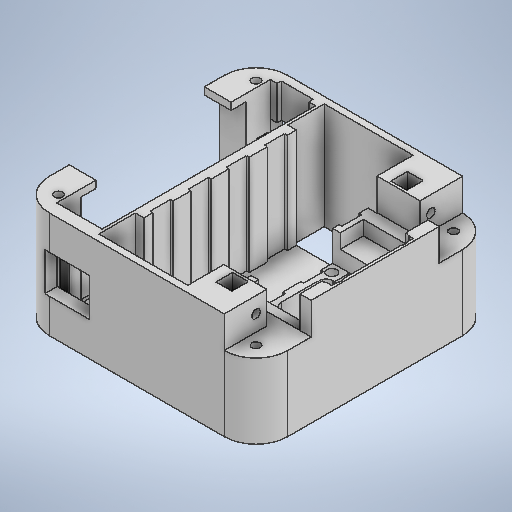
# Autodesk Inventor part: enclosure
Saved by Autodesk Inventor 2025 (Build 290162000, 162)
## iProperties
Created: 2025-10-18
Part Number: enclosure
Material: 一般
Document SubType Name: Modeling
Designer: sooo1
Density: 1 g/cm^3
Appearance: 既定
Author: sooo1
Autodesk Inventor part; units mm, degrees
ref_plane "YZ Plane" through (0, 0, 0) normal (1, 0, 0) x (0, 1, 0)
ref_plane "XZ Plane" through (0, 0, 0) normal (0, 1, 0) x (-1, 0, 0)
sketch "スケッチ1" plane through (0, 0, 0) normal (0, 1, 0) x (-1, 0, 0)
  line L0 (37.55, 37.55) -> (-37.55, 37.55)
  line L1 (-37.55, 37.55) -> (-37.55, -37.55)
  line L2 (-37.55, -37.55) -> (37.55, -37.55)
  line L3 (37.55, -37.55) -> (37.55, 37.55)
  line L4 (37.55, 37.55) -> (-37.55, -37.55) construction
  line L5 (-37.55, 37.55) -> (37.55, -37.55) construction
  line L6 (36.55, 36.55) -> (-36.55, 36.55)
  line L7 (-36.55, 36.55) -> (-36.55, -36.55)
  line L8 (-36.55, -36.55) -> (36.55, -36.55)
  line L9 (36.55, -36.55) -> (36.55, 36.55)
  line L10 (52.57, 0) -> (-52.57, 0) construction
  line L11 (0, -52.57) -> (0, 52.57) construction
  line L12 (14, -25) -> (-14, -25)
  line L13 (-14, -25) -> (-14, -35.5)
  line L14 (-14, -35.5) -> (14, -35.5)
  line L15 (14, -35.5) -> (14, -25)
  line L16 (14, -25) -> (-14, -35.5) construction
  line L17 (-14, -25) -> (14, -35.5) construction
  line L18 (0, 37.55) -> (0, -37.55) construction
  circle A0 centre (-13.68, -10.17) radius 1.6
  line L19 (14, -30.25) -> (-14, -30.25) construction
  line L20 (-11.15, 0) -> (-11.15, -24)
  line L21 (11.15, -24) -> (11.15, 0)
  line L22 (-11.15, 12.7) -> (-36.55, 12.7)
  line L23 (-36.55, 12.7) -> (-36.55, -12.7) construction
  line L24 (-36.55, -12.7) -> (-11.15, -12.7)
  line L25 (-11.15, -12.7) -> (-11.15, 12.7) construction
  line L26 (-11.15, 12.7) -> (-36.55, -12.7) construction
  line L27 (-36.55, 12.7) -> (-11.15, -12.7) construction
  line L28 (-13.68, 10.17) -> (-34.02, 10.17) construction
  line L29 (-34.02, 10.17) -> (-34.02, -10.17) construction
  line L30 (-34.02, -10.17) -> (-13.68, -10.17) construction
  line L31 (-13.68, -10.17) -> (-13.68, 10.17) construction
  line L32 (-13.68, 10.17) -> (-34.02, -10.17) construction
  line L33 (-34.02, 10.17) -> (-13.68, -10.17) construction
  circle A1 centre (-13.68, 10.17) radius 1.6
  circle A2 centre (-34.02, 10.17) radius 1.6
  circle A3 centre (-34.02, -10.17) radius 1.6
  line L34 (11.15, 0) -> (-11.15, 0) construction
  line L35 (11.15, -24) -> (-11.15, -24)
  line L36 (8.8, -24) -> (-8.8, -24) construction
  line L37 (-8.8, -24) -> (-8.8, -27)
  line L38 (-8.8, -27) -> (8.8, -27)
  line L39 (8.8, -27) -> (8.8, -24)
  line L40 (8.8, -24) -> (-8.8, -27) construction
  line L41 (-8.8, -24) -> (8.8, -27) construction
  line L42 (11.15, -3) -> (12, -3)
  line L43 (12, -3) -> (12, -9)
  line L44 (12, -9) -> (11.15, -9)
  line L45 (11.15, -12) -> (-11.15, -12) construction
  line L46 (12, -6) -> (-12, -6) construction
  line L47 (11.15, -21) -> (12, -21)
  line L48 (12, -21) -> (12, -15)
  line L49 (12, -15) -> (11.15, -15)
  line L50 (-11.15, -3) -> (-12, -3)
  line L51 (-12, -3) -> (-12, -9)
  line L52 (-12, -9) -> (-11.15, -9)
  line L53 (-12, -15) -> (-11.15, -15)
  line L54 (-12, -21) -> (-12, -15)
  line L55 (-11.15, -21) -> (-12, -21)
  line L56 (14, 25) -> (-14, 25)
  line L57 (-14, 25) -> (-14, 35.5)
  line L58 (-14, 35.5) -> (14, 35.5)
  line L59 (14, 35.5) -> (14, 25)
  line L60 (-11.15, 0) -> (-11.15, 24)
  line L61 (11.15, 24) -> (11.15, 0)
  line L62 (11.15, 24) -> (-11.15, 24)
  line L63 (8.8, 24) -> (-8.8, 24) construction
  line L64 (-8.8, 24) -> (-8.8, 27)
  line L65 (-8.8, 27) -> (8.8, 27)
  line L66 (8.8, 27) -> (8.8, 24)
  line L67 (11.15, 3) -> (12, 3)
  line L68 (12, 3) -> (12, 9)
  line L69 (12, 9) -> (11.15, 9)
  line L70 (12, 15) -> (11.15, 15)
  line L71 (12, 21) -> (12, 15)
  line L72 (11.15, 21) -> (12, 21)
  line L73 (-12, 3) -> (-12, 9)
  line L74 (-11.15, 3) -> (-12, 3)
  line L75 (-12, 9) -> (-11.15, 9)
  line L76 (-12, 21) -> (-12, 15)
  line L77 (-12, 15) -> (-11.15, 15)
  line L78 (-11.15, 21) -> (-12, 21)
  line L79 (15, 33.5) -> (29, 33.5)
  line L80 (29, 33.5) -> (29, -33.5)
  line L81 (29, -33.5) -> (15, -33.5)
  line L82 (15, -33.5) -> (15, 33.5)
  line L83 (15, 33.5) -> (29, -33.5) construction
  line L84 (29, 33.5) -> (15, -33.5) construction
  line L85 (-33.85, 20) -> (-13.85, 20)
  line L86 (-13.85, 20) -> (-13.85, -20)
  line L87 (-13.85, -20) -> (-33.85, -20)
  line L88 (-33.85, -20) -> (-33.85, 20)
  line L89 (-33.85, 20) -> (-13.85, -20) construction
  line L90 (-13.85, 20) -> (-33.85, -20) construction
  line L91 (37.55, 25.5) -> (15, 25.5) construction
  circle A4 centre (-21, -30.25) radius 3.1
  line L92 (-21, -37.55) -> (-21, 37.55) construction
  circle A5 centre (-21, 30.25) radius 3.1
  circle A6 centre (21, -30.25) radius 3.1
  circle A7 centre (21, 30.25) radius 3.1
  circle A8 centre (-21, -30.25) radius 4.1
  circle A9 centre (-21, 30.25) radius 4.1
  circle A10 centre (21, -30.25) radius 4.1
  circle A11 centre (21, 30.25) radius 4.1
  circle A12 centre (33, 0) radius 2.6
  circle A13 centre (33, 0) radius 3.5
  circle A14 centre (-33, 0) radius 2.6
  circle A15 centre (-33, 0) radius 3.5
  line L93 (-27.85, 4) -> (-19.85, 4)
  line L94 (-19.85, 4) -> (-19.85, -4)
  line L95 (-19.85, -4) -> (-27.85, -4)
  line L96 (-27.85, -4) -> (-27.85, 4)
  line L97 (-27.85, 4) -> (-19.85, -4) construction
  line L98 (-19.85, 4) -> (-27.85, -4) construction
  line L99 (26, -34) -> (18, -34)
  line L100 (18, -34) -> (18, -33.5)
  line L101 (18, -33.5) -> (26, -33.5) construction
  line L102 (26, -33.5) -> (26, -34)
  line L103 (26, -34) -> (18, -33.5) construction
  line L104 (18, -34) -> (26, -33.5) construction
  line L105 (22, -33.5) -> (22, 33.5) construction
  line L106 (-11.15, 24) -> (-11.15, 25)
  line L107 (11.15, 24) -> (11.15, 25)
  line L108 (11.15, -24) -> (11.15, -25)
  line L109 (-11.15, -24) -> (-11.15, -25)
  line L110 (14, 25) -> (14, 24)
  line L111 (14, 24) -> (11.15, 24)
  line L112 (-11.15, 24) -> (-14, 24)
  line L113 (-14, 24) -> (-14, 25)
  line L114 (14, -25) -> (14, -24)
  line L115 (14, -24) -> (11.15, -24)
  line L116 (-11.15, -24) -> (-14, -24)
  line L117 (-14, -24) -> (-14, -25)
  line L118 (-11.15, 8.17) -> (-36.55, 8.17)
  line L119 (-11.15, -8.17) -> (-36.55, -8.17)
  line L120 (-11.15, 13) -> (-36.55, 13)
  line L121 (-11.15, -13) -> (-36.55, -13)
  line L122 (-16.65, 13) -> (-16.65, -13)
  line L123 (-29.55, 13) -> (-29.55, -13)
  line L124 (-36.55, 13) -> (-37.55, 13)
  line L125 (-36.55, -13) -> (-37.55, -13)
  line L126 (-27.85, 4) -> (-27.85, 13)
  line L127 (-27.85, -4) -> (-27.85, -13)
  point P0 (0, 0)
  point P1 (0, -30.25)
  point P2 (-23.85, 0)
  point P3 (0, -25.5)
  point P4 (0, 0)
  point P5 (0, -6)
  point P6 (-12, 6)
  point P7 (12, 6)
  point P8 (22, 0)
  point P9 (-23.85, 0)
  point P10 (22, -33.75)
  point P11 (-29.55, 0.5895)
  point P12 (-29.55, -0.5895)
  point P13 (-29.55, -8.17)
  point P14 (-29.55, 8.17)
  point P15 (-27.85, 12.7)
  point P16 (-29.55, 12.7)
  point P17 (-16.65, -8.17)
  point P18 (-13.85, -8.17)
  point P19 (-13.85, 8.17)
  point P20 (-16.65, 8.17)
  point P21 (-33.85, 8.17)
  point P22 (-33.85, -8.17)
  point P23 (-29.55, -12.7)
  point P24 (-16.65, -12.7)
  point P25 (-16.65, 12.7)
  dimension "d1" = 1
  dimension "d2" = 10.5
  dimension "d3" = 28
  dimension "d5" = 3.2
  dimension "d11" = 25.4
  dimension "d12" = 20.34
  dimension "d15" = 360
  dimension "d18" = 22.3
  dimension "d19" = 17.6
  dimension "d20" = 27
  dimension "d21" = 24
  dimension "d22" = 1
  dimension "d25" = 24
  dimension "d26" = 12
  dimension "d27" = 6
  dimension "d32" = 67
  dimension "d33" = 14
  dimension "d34" = 1
  dimension "d35" = 40
  dimension "d36" = 20
  dimension "d41" = 8
  dimension "d47" = 6.2
  dimension "d48" = 7
  dimension "d49" = 1
  dimension "d54" = 5.2
  dimension "d55" = 7
  dimension "d56" = 33
  dimension "d86" = 8
  dimension "d110" = 8
  dimension "d111" = 0.5
  dimension "d177" = 8.17
  dimension "d178" = 8.17
  dimension "d179" = 0.3
  dimension "d180" = 0.3
  dimension "d181" = 7
  dimension "d182" = 5.5
  constraints: 252 end point, 48 symmetric about line, 45 point on line, 31 perpendicular, 30 midpoint, 22 parallel, 16 centre point, 11 horizontal, 8 collinear, 5 coincident, 3 equal length, 1 vertical, 20 other
  measures "d1" distance between parallel lines of L0 L6
  measures "d2" distance of L14.end L12.start
  measures "d3" distance of L13.end L14.end
  measures "d5" diameter of A0
  measures "d11" distance of L24.end L22.start
  measures "d12" distance of L30.end L28.start
  measures "d18" distance between parallel lines of L20 L21
  measures "d19" distance of L37.end L38.end
  measures "d20" distance between parallel lines of L34 L38
  measures "d21" distance of L21.start L21.end
  measures "d22" distance between parallel lines of L12 L35
  measures "d25" distance of L46.start L46.end
  measures "d26" diameter of L46 L45
  measures "d27" distance of L42.end L43.end
  measures "d32" distance of L79.end L80.end
  measures "d33" distance of L79.start L79.end
  measures "d34" distance between parallel lines of L82 L59
  measures "d35" distance of L87.end L85.start
  measures "d36" distance of L85.start L85.end
  measures "d41" distance between parallel lines of L79 L91
  measures "d47" diameter of A4
  measures "d48" distance between parallel lines of L13 L92
  measures "d49" radial gap between concentric circles of A4 A8
  measures "d54" diameter of A12
  measures "d55" diameter of A13
  measures "d56" distance from line of L11 A12.centre
  measures "d86" distance of L95.end L93.start
  measures "d110" distance of L99.start L99.end
  measures "d111" distance of L101.end L99.start
  measures "d177" distance between parallel lines of L10 L118
  measures "d178" distance between parallel lines of L119 L10
  measures "d179" distance between parallel lines of L22 L120
  measures "d180" distance between parallel lines of L121 L24
  measures "d181" distance between parallel lines of L23 L123
  measures "d182" distance between parallel lines of L25 L122
extrude "押し出し3" add sketch "スケッチ1" along normal blind 33.5 contours L3 L2 L1 L125 L7 L8 L9 L6 L124 L0 | L124 L7 L125 L1 | L120 L88 L22 L7 | L7 L6 L9 L8 L121 L88 L87 L86 L20 L53 L54 L55 L116 L117 L13 L14 L15 L114 L115 L21 L47 L48 L49 L44 L43 L42 L61 L67 L68 L69 L70 L71 L72 L111 L110 L59 L58 L57 L113 L112 L60 L78 L76 L77 L120 L85 | L7 L24 L88 L121 | L22 L88 A2 L118 L7 | L120 L123 L22 L88 | L88 L85 L86 L120 | L7 L119 L88 A3 L24 | L121 L86 L87 L88 | L88 L24 L123 L121 | L118 L88 A15 L119 L7 | L22 L123 L118 L88 A2 | L120 L126 L22 L123 | L88 A3 L119 L123 L24 | L123 L24 L127 L121 | L118 L123 A15 L88 | L22 L126 L118 L123 | L88 A2 | A2 L88 | L120 L122 L22 L126 | L88 A15 L123 L119 | L123 L119 L127 L24 | L88 A3 | A3 L88 | L127 L24 L122 L121 | A15 L123 L88 A14 | L88 A14 A15 | L118 L126 L96 L127 L119 L123 A15 | L22 L122 L118 L126 | L120 L60 L22 L86 | L86 L22 L122 L120 | L127 L119 L122 L24 | L121 L122 L24 L86 | L86 L24 L20 L121 | A14 L88 | L88 A14 | A15 L123 | L118 L122 L119 L127 L95 L94 L93 L126 | L22 L86 A1 L118 L122 | L22 L60 L75 L73 L118 L86 A1 | L60 L62 L61 L21 L35 L20 | L122 L119 L86 A0 L24 | L86 A0 L119 L51 L52 L20 L24 | L118 L86 L119 L122 | L93 L94 L95 L96 | L86 A1 | A1 L86 | L77 L76 L78 L60 | L86 A0 | A0 L86 | L20 L55 L54 L53 | L118 L73 L74 L60 L20 L50 L51 L119 L86 | L60 L118 L73 L75 | L52 L51 L119 L20 | L118 L60 L74 L73 | L106 L56 L64 L62 | L112 L113 L56 L106 | L51 L50 L20 L119 | L35 L37 L12 L109 | L109 L12 L117 L116 | L64 L56 L66 L62 | L56 L57 L58 L59 L66 L65 L64 | L35 L39 L12 L37 | L12 L37 L38 L39 L15 L14 L13 | L66 L56 L107 L62 | L64 L65 L66 L56 | L35 L108 L12 L39 | L12 L39 L38 L37 | L107 L56 L110 L111 | L115 L114 L12 L108 | L72 L71 L70 L61 | L21 L49 L48 L47 | L69 L68 L67 L61 | L21 L42 L43 L44 | L79 A11 L80 L81 A10 L82 | A11 L79 | L79 A11 | L81 A10 L99 L100 | A10 L81 | L81 A10 L99 | L81 L102 L99 A10 | L99 A10 | A4 | A5 | A6 | A7 | A8 | A9 | A12 | A13
fillet "フィレット1" radius 10 4 edges at (37.55, 16.75, 37.55) (37.55, 16.75, -37.55) (-37.55, 16.75, -37.55) (-37.55, 16.75, 37.55)
extrude "押し出し11" cut sketch "スケッチ1" along normal through all contours L56 L57 L58 L59 L66 L65 L64 | L12 L37 L38 L39 L15 L14 L13 | L64 L65 L66 L56 | L12 L39 L38 L37
extrude "押し出し12" cut sketch "スケッチ1" along normal blind 1.5 contours A4 | A5 | A6 | A7
extrude "押し出し13" cut sketch "スケッチ1" along normal blind 1.5 contours A14 L88 | L88 A14 | A12
sketch "スケッチ5" plane through (0, 0, 0) normal (0, 1, 0) x (-1, 0, 0)
  line L0 (-12, 9) -> (-11.15, 9) projected
  line L1 (-11.15, 0) -> (-11.15, 24) projected
  line L2 (-12, 3) -> (-12, 9) projected
  line L3 (-11.15, 3) -> (-12, 3) projected
  line L4 (-12, 15) -> (-11.15, 15) projected
  line L5 (-12, 21) -> (-12, 15) projected
  line L6 (11.15, 3) -> (12, 3) projected
  line L7 (-11.15, 21) -> (-12, 21) projected
  line L8 (11.15, 21) -> (12, 21) projected
  line L9 (11.15, 24) -> (-11.15, 24) projected
  line L10 (-8.8, 24) -> (-8.8, 27) projected
  line L11 (8.8, 24) -> (-8.8, 24) construction
  line L12 (8.8, 27) -> (8.8, 24) projected
  line L13 (-8.8, 27) -> (8.8, 27) projected
  line L14 (11.15, 0) -> (-11.15, 0) construction
  line L15 (11.15, -12) -> (-11.15, -12) construction
  line L16 (12, -9) -> (11.15, -9) projected
  line L17 (11.15, -3) -> (12, -3) projected
  line L18 (12, -3) -> (12, -9) projected
  line L19 (12, -6) -> (-12, -6) construction
  line L20 (-12, -9) -> (-11.15, -9) projected
  line L21 (-12, -3) -> (-12, -9) projected
  line L22 (-11.15, -3) -> (-12, -3) projected
  line L23 (-11.15, -12.7) -> (-11.15, 12.7) construction
  line L24 (-11.15, 0) -> (-11.15, -24) projected
  line L25 (11.15, -24) -> (11.15, 0) projected
  line L26 (12, -15) -> (11.15, -15) projected
  line L27 (12, -21) -> (12, -15) projected
  line L28 (12, 9) -> (11.15, 9) projected
  line L29 (12, 3) -> (12, 9) projected
  line L30 (12, 15) -> (11.15, 15) projected
  line L31 (12, 21) -> (12, 15) projected
  line L32 (11.15, 24) -> (11.15, 0) projected
  line L33 (11.15, -24) -> (-11.15, -24) projected
  line L34 (8.8, -24) -> (-8.8, -24) construction
  line L35 (-12, -15) -> (-11.15, -15) projected
  line L36 (-12, -21) -> (-12, -15) projected
  line L37 (-11.15, -21) -> (-12, -21) projected
  line L38 (11.15, -21) -> (12, -21) projected
  line L39 (-8.8, -27) -> (8.8, -27) projected
  line L40 (-8.8, -24) -> (-8.8, -27) projected
  line L41 (8.8, -27) -> (8.8, -24) projected
  line L42 (-11.15, -14.85) -> (-12.15, -14.85)
  line L43 (-12.15, -14.85) -> (-12.15, -21.15)
  line L44 (-12.15, -21.15) -> (-11.15, -21.15)
  line L45 (-11.15, -9.15) -> (-12.15, -9.15)
  line L46 (-12.15, -9.15) -> (-12.15, -2.85)
  line L47 (-12.15, -2.85) -> (-11.15, -2.85)
  line L48 (11.15, -14.85) -> (12.15, -14.85)
  line L49 (12.15, -14.85) -> (12.15, -21.15)
  line L50 (12.15, -21.15) -> (11.15, -21.15)
  line L51 (11.15, -9.15) -> (12.15, -9.15)
  line L52 (12.15, -9.15) -> (12.15, -2.85)
  line L53 (12.15, -2.85) -> (11.15, -2.85)
  line L54 (-11.15, 9.15) -> (-12.15, 9.15)
  line L55 (-12.15, 9.15) -> (-12.15, 2.85)
  line L56 (-12.15, 2.85) -> (-11.15, 2.85)
  line L57 (-11.15, 14.85) -> (-12.15, 14.85)
  line L58 (-12.15, 14.85) -> (-12.15, 21.15)
  line L59 (-12.15, 21.15) -> (-11.15, 21.15)
  line L60 (11.15, 14.85) -> (12.15, 14.85)
  line L61 (12.15, 14.85) -> (12.15, 21.15)
  line L62 (12.15, 21.15) -> (11.15, 21.15)
  line L63 (-11.3, -24.15) -> (-11.3, 0)
  line L64 (-11.3, 0) -> (-11.3, 24.15)
  line L65 (-11.3, 24.15) -> (11.3, 24.15)
  line L66 (11.3, 24.15) -> (11.3, 0)
  line L67 (11.3, 0) -> (11.3, -24.15)
  line L68 (11.3, -24.15) -> (-11.3, -24.15)
  line L69 (8.95, 27.15) -> (8.95, 23.85)
  line L70 (8.95, 23.85) -> (-8.95, 23.85)
  line L71 (-8.95, 23.85) -> (-8.95, 27.15)
  line L72 (-8.95, 27.15) -> (8.95, 27.15)
  line L73 (8.95, -27.15) -> (-8.95, -27.15)
  line L74 (-8.95, -27.15) -> (-8.95, -23.85)
  line L75 (-8.95, -23.85) -> (8.95, -23.85)
  line L76 (8.95, -23.85) -> (8.95, -27.15)
  line L77 (11.15, 9.15) -> (12.15, 9.15)
  line L78 (12.15, 9.15) -> (12.15, 2.85)
  line L79 (12.15, 2.85) -> (11.15, 2.85)
  point P0 (0, 0)
  point P1 (0, 0)
  point P2 (-12, 6)
  point P3 (12, 6)
  point P4 (0, -6)
  point P5 (0, 0)
  point P6 (-11.3, -14.85)
  point P7 (-11.3, -21.15)
  point P8 (-8.95, -24.15)
  point P9 (8.95, -24.15)
  point P10 (11.3, -21.15)
  point P11 (11.3, -14.85)
  point P12 (11.3, -9.15)
  point P13 (11.3, -2.85)
  point P14 (11.3, 2.85)
  point P15 (11.3, 9.15)
  point P16 (11.3, 14.85)
  point P17 (11.3, 21.15)
  point P18 (8.95, 24.15)
  point P19 (-8.95, 24.15)
  point P20 (-11.3, 21.15)
  point P21 (-11.3, 14.85)
  point P22 (-11.3, 9.15)
  point P23 (-11.3, 2.85)
  point P24 (-11.3, -2.85)
  point P25 (-11.3, -9.15)
  dimension "d73" = 0.15
  dimension "d74" = 0.15
  dimension "d75" = 0.15
  dimension "d76" = 0.15
  dimension "d77" = 0.15
  dimension "d78" = 0.15
  dimension "d79" = 0.15
  dimension "d80" = 0.15
  dimension "d81" = 0.15
  dimension "d82" = 0.15
  dimension "d83" = 0.15
  constraints: 76 end point, 27 other
  measures "d73" distance between parallel lines of L24 L63
  measures "d74" distance between parallel lines of L36 L43
  measures "d75" distance between parallel lines of L39 L73
  measures "d76" distance between parallel lines of L21 L46
  measures "d77" distance between parallel lines of L2 L55
  measures "d78" distance between parallel lines of L5 L58
  measures "d79" distance between parallel lines of L13 L72
  measures "d80" distance between parallel lines of L61 L31
  measures "d81" distance between parallel lines of L18 L52
  measures "d82" distance between parallel lines of L27 L49
  measures "d83" distance between parallel lines of L29 L78
extrude "押し出し14" cut sketch "スケッチ5" against normal blind 31.5 from surface at 33.5
sketch "スケッチ6" plane through (0, 0, 0) normal (0, 1, 0) x (-1, 0, 0)
  line L0 (-11.15, 12.7) -> (-36.55, 12.7) projected
  circle A0 centre (-13.68, 10.17) radius 1.6 projected
  line L1 (-11.15, 0) -> (-11.15, 24) projected
  line L2 (-11.15, 0) -> (-11.15, -24) projected
  line L3 (-36.55, -12.7) -> (-11.15, -12.7) projected
  line L4 (-36.55, 12.7) -> (-36.55, -12.7) projected
  circle A1 centre (-34.02, -10.17) radius 1.6 projected
  circle A2 centre (-34.02, 10.17) radius 1.6 projected
  circle A3 centre (-13.68, -10.17) radius 1.6 projected
  line L5 (-11.15, 12.85) -> (-36.7, 12.85)
  line L6 (-36.7, 12.85) -> (-36.7, -12.85)
  line L7 (-36.7, -12.85) -> (-11.15, -12.85)
  circle A4 centre (-13.68, 10.17) radius 3
  circle A5 centre (-34.02, 10.17) radius 3
  circle A6 centre (-13.68, -10.17) radius 3
  circle A7 centre (-34.02, -10.17) radius 3
  line L8 (-11.15, 12.85) -> (-11.15, -12.85)
  line L9 (-12, 9) -> (-11.15, 9) projected
  line L10 (-11.15, 3) -> (-12, 3) projected
  line L11 (-11.15, -3) -> (-12, -3) projected
  line L12 (-12, -9) -> (-11.15, -9) projected
  line L13 (-11.15, -12.7) -> (-11.15, 12.7) projected
  line L14 (-36.55, 36.55) -> (-36.55, -36.55) projected
  line L15 (-36.55, 12.7) -> (-36.55, 12.85)
  line L16 (-36.55, -12.7) -> (-37.55, -12.85)
  line L17 (-37.55, 27.55) -> (-37.55, -27.55) projected
  line L18 (-11.15, -8.17) -> (-36.55, -8.17) projected
  line L19 (-11.15, 8.17) -> (-36.55, 8.17) projected
  line L20 (-36.55, 8.17) -> (-36.7, 8.17)
  line L21 (-36.55, -8.17) -> (-36.7, -8.17)
  point P0 (0, 0)
  point P1 (-36.7, -11.5182)
  point P2 (-36.7, -8.8218)
  point P3 (-32.6718, -12.85)
  point P4 (-35.3682, -12.85)
  point P5 (-36.7, 8.8218)
  point P6 (-36.7, 11.5182)
  point P7 (-35.3682, 12.85)
  point P8 (-32.6718, 12.85)
  point P9 (-36.55, -12.85)
  point P10 (-36.55, -11.7822)
  point P11 (-35.6322, -12.7)
  point P12 (-36.55, -12.7)
  point P13 (-36.4, -10.6381)
  point P14 (-36.4, -9.7019)
  point P15 (-36.4, 9.7019)
  point P16 (-36.4, 10.6381)
  point P17 (-36.55, 12.7)
  point P18 (-35.6322, 12.7)
  point P19 (-36.55, 11.7822)
  dimension "d89" = 0.15
  dimension "d92" = 6
  constraints: 14 end point, 6 point on line, 4 centre point, 3 equal radius, 3 perpendicular, 1 horizontal, 9 other
  measures "d89" distance between parallel lines of L0 L5
  measures "d92" diameter of A4
extrude "押し出し16" cut sketch "スケッチ6" against normal blind 19.5 from surface at 33.5 contours L1 A4 L0 | L0 A4 L5 L1 | A4 L1 L19 L0 | L0 A4 L5 | A4 L19 A5 L0 | L0 A5 L5 A4 | A5 L19 L4 L0 | L0 A5 L5 | L19 A4 | A4 L19 L1 L2 L18 A6 A7 L4 A5 | L1 L19 A4 | A5 L4 L0 | L0 L14 L5 A5 | L5 A5 | A5 L19 | L4 A5 L6 L5 L14 | L4 A5 L6 | L19 L4 A5 | L4 L20 L6 A5 | L6 A5 | L4 L21 L6 L20 | L18 A7 L4 | L4 A7 L6 L21 | A7 L18 L3 L4 | L4 A7 L6 | A7 L18 | L2 A6 L18 | A7 L3 L4 | L4 L16 L6 A7 | L6 A7 | L18 A6 L3 A7 | L2 A6 L3 L18 | L18 A6 | L3 A7 L7 L14 | L14 L7 L6 L16 | L3 A7 L7 | L3 A6 L7 A7 | L7 A7 | L3 A6 L7 | L2 L3 A6 | L3 L2 L7 A6 | A0 | A1 | A2 | A3
extrude "押し出し15" cut sketch "スケッチ1" along normal through all contours L88 A2 | A2 L88 | L88 A3 | A3 L88 | L93 L94 L95 L96 | L86 A1 | A1 L86 | L86 A0 | A0 L86
extrude "押し出し17" cut sketch "スケッチ6" along normal blind 4 contours A5 L19 L4 L0 | L0 A5 L5 | L5 A5 | A5 L19 | L4 A5 L6 | L6 A5 | A7 L18 L3 L4 | L4 A7 L6 | A7 L18 | L6 A7 | L3 A7 L7 | L7 A7 | A1 | A2
sketch "スケッチ7" plane through (0, 0, 0) normal (0, 1, 0) x (-1, 0, 0)
  line L0 (-33.85, 20) -> (-13.85, 20) projected
  line L1 (-13.85, 20) -> (-13.85, -20) projected
  line L2 (-33.85, -20) -> (-33.85, 20) projected
  line L3 (-13.85, -20) -> (-33.85, -20) projected
  line L4 (-13.7, 20.15) -> (-34, 20.15)
  line L5 (-34, 20.15) -> (-34, -20.15)
  line L6 (-34, -20.15) -> (-13.7, -20.15)
  line L7 (-13.7, -20.15) -> (-13.7, 20.15)
  point P0 (0, 0)
  dimension "d95" = 0.15
  constraints: 8 end point, 3 other
  measures "d95" distance between parallel lines of L0 L4
extrude "押し出し18" cut sketch "スケッチ7" against normal blind 14.5 from surface at 33.5 contours L0 L1 L3 L2 | L7 L6 L5 L4
sketch "スケッチ9" plane through (0, 0, 0) normal (0, 1, 0) x (-1, 0, 0)
  line L0 (29, 33.5) -> (29, -33.5) projected
  line L1 (29, -33.5) -> (15, -33.5) projected
  line L2 (15, -33.5) -> (15, 33.5) projected
  line L3 (15, 33.5) -> (29, 33.5) projected
  line L4 (29.15, -33.65) -> (29.15, 33.65)
  line L5 (29.15, 33.65) -> (14.85, 33.65)
  line L6 (14.85, 33.65) -> (14.85, -33.65)
  line L7 (14.85, -33.65) -> (29.15, -33.65)
  line L8 (15, -33.5) -> (15, -33.65)
  line L9 (15, 33.5) -> (15, 33.65)
  line L10 (26, -33.5) -> (26, -34) projected
  line L11 (26, -34) -> (18, -34) projected
  line L12 (18, -34) -> (18, -33.5) projected
  line L13 (16, -33.5) -> (16, -36)
  line L14 (16, -36) -> (28, -36)
  line L15 (28, -36) -> (28, -33.5)
  line L16 (28, -36) -> (28, -39.9042)
  line L17 (28, -39.9042) -> (16, -39.9042)
  line L18 (16, -39.9042) -> (16, -36)
  line L19 (17, -33.5) -> (17, -35)
  line L20 (17, -35) -> (27, -35)
  line L21 (27, -35) -> (27, -33.5)
  point P0 (0, 0)
  point P1 (22, -33.5)
  point P2 (18, -33.65)
  point P3 (26, -33.65)
  point P4 (17, -33.65)
  point P5 (27, -33.65)
  dimension "d109" = 0.15
  dimension "d113" = 12
  dimension "d116" = 10
  constraints: 30 end point, 3 point on line, 2 perpendicular, 2 vertical, 1 midpoint, 7 other
  measures "d109" distance from line of point (22, -33.5) L7
  measures "d113" distance of L13.end L14.end
  measures "d116" distance of L19.end L20.end
extrude "押し出し21" cut sketch "スケッチ9" against normal blind 31.25 from surface at 33.5 contours L3 L9 L5 L4 L7 L15 L1 L0 | L0 L1 L2 L3 | L2 L8 L7 L6 L5 L9 | L15 L7 L21 L1 | L1 L13 L7 L8 | L21 L7 L10 L1 | L1 L19 L7 L13 | L10 L7 L12 L1 | L21 L20 L19 L7 L12 L11 L10 | L1 L12 L7 L19 | L10 L11 L12 L7
sketch "スケッチ8" plane through (0, 0, 0) normal (1, 0, 0) x (0, 1, 0)
  line L0 (-10.4294, 0) -> (62.5761, 0) construction
  line L1 (0, -52.2157) -> (0, 71.794) construction
  line L2 (30.25, -33.5) -> (3.25, -33.5)
  line L3 (3.25, -33.5) -> (3.25, 33.5)
  line L4 (3.25, 33.5) -> (30.25, 33.5)
  line L5 (30.25, 33.5) -> (30.25, -33.5)
  line L6 (30.25, -33.5) -> (3.25, 33.5) construction
  line L7 (3.25, -33.5) -> (30.25, 33.5) construction
  line L8 (31.25, -34.5) -> (2.25, -34.5)
  line L9 (2.25, -34.5) -> (2.25, 34.5)
  line L10 (2.25, 34.5) -> (31.25, 34.5)
  line L11 (31.25, 34.5) -> (31.25, -34.5)
  line L12 (20.75, 33.5) -> (12.75, 33.5) construction
  line L13 (12.75, 33.5) -> (12.75, 34)
  line L14 (12.75, 34) -> (20.75, 34)
  line L15 (20.75, 34) -> (20.75, 33.5)
  line L16 (20.75, 33.5) -> (12.75, 34) construction
  line L17 (12.75, 33.5) -> (20.75, 34) construction
  line L18 (16.75, -33.5) -> (16.75, 33.5) construction
  line L19 (52.1468, -21.2895) -> (31.25, -21.2895)
  line L20 (31.25, -21.2895) -> (31.25, 21.2895) construction
  line L21 (31.25, 21.2895) -> (52.1468, 21.2895)
  line L22 (52.1468, 21.2895) -> (52.1468, -21.2895)
  line L23 (52.1468, -21.2895) -> (31.25, 21.2895) construction
  line L24 (31.25, -21.2895) -> (52.1468, 21.2895) construction
  line L25 (22.75, 33.5) -> (10.75, 33.5) construction
  line L26 (10.75, 33.5) -> (10.75, 54.0784)
  line L27 (10.75, 54.0784) -> (22.75, 54.0784)
  line L28 (22.75, 54.0784) -> (22.75, 33.5)
  line L29 (22.75, 33.5) -> (10.75, 54.0784) construction
  line L30 (10.75, 33.5) -> (22.75, 54.0784) construction
  line L31 (31.25, -26) -> (2.25, -26)
  line L32 (31.25, 26) -> (2.25, 26)
  point P0 (0, 0)
  point P1 (16.75, 0)
  point P2 (16.75, 33.75)
  point P3 (41.6984, 0)
  point P4 (16.75, 43.7892)
  point P5 (10.75, 34.5)
  point P6 (22.75, 34.5)
  point P7 (30.25, 26)
  point P8 (3.25, 26)
  point P9 (3.25, -26)
  point P10 (30.25, -26)
  dimension "d98" = 27
  dimension "d99" = 67
  dimension "d100" = 1
  dimension "d101" = 0.5
  dimension "d102" = 8
  dimension "d103" = 16.75
  dimension "d106" = 12
  dimension "d117" = 26
  constraints: 62 end point, 10 midpoint, 10 parallel, 7 perpendicular, 6 point on line, 4 horizontal, 3 collinear, 2 symmetric about line, 3 other
  measures "d98" distance of L2.start L2.end
  measures "d99" distance of L4.end L2.start
  measures "d100" distance between parallel lines of L2 L8
  measures "d101" distance of L14.end L12.start
  measures "d102" distance of L13.end L14.end
  measures "d103" distance between parallel lines of L1 L18
  measures "d106" distance of L26.end L27.end
  measures "d117" distance between parallel lines of L31 L0
extrude "押し出し22" cut sketch "スケッチ8" against normal blind 31.25 from surface at -29.15 contours L31 L3 L32 L5 | L5 L32 L11 L31 | L11 L21 L22 L19
sketch "スケッチ10" plane through (0, 0, 0) normal (0, 0, 1) x (1, 0, 0)
  line L0 (-15, 22.75) -> (-29, 22.75)
  line L1 (-29, 22.75) -> (-29, 10.75)
  line L2 (-29, 10.75) -> (-15, 10.75)
  line L3 (-15, 10.75) -> (-15, 22.75)
  line L4 (-15, 22.75) -> (-29, 10.75) construction
  line L5 (-29, 22.75) -> (-15, 10.75) construction
  line L6 (-34.8, 0) -> (5.8, 0) construction
  point P0 (0, 0)
  point P1 (-15, 0)
  point P2 (-15, 0)
  point P3 (-15, 0)
  point P4 (-22, 16.75)
  dimension "d120" = 14
  dimension "d121" = 12
  dimension "d122" = 16.75
  dimension "d123" = 7
  constraints: 12 end point, 2 midpoint, 2 parallel, 1 horizontal, 1 perpendicular
  measures "d120" distance of L0.start L0.end
  measures "d121" distance of L2.end L0.start
  measures "d122" distance from line of L6 point (-22, 16.75)
  measures "d123" horizontal distance of point (-22, 16.75) point (-15, 0)
extrude "押し出し23" cut sketch "スケッチ10" along normal through all both and the other way through all
sketch "スケッチ11" plane through (0, 0, 0) normal (0, 1, 0) x (-1, 0, 0)
  circle A0 centre (31.1127, 31.1127) radius 1.35
  line L0 (37.55, 37.55) -> (-37.55, -37.55) construction
  line L1 (-37.55, 37.55) -> (37.55, -37.55) construction
  circle A1 centre (0, 0) radius 44 construction
  circle A2 centre (-31.1127, 31.1127) radius 1.35
  circle A3 centre (-31.1127, -31.1127) radius 1.35
  circle A4 centre (31.1127, -31.1127) radius 1.35
  circle A5 centre (31.1127, 31.1127) radius 2.5
  circle A6 centre (-31.1127, 31.1127) radius 2.5
  circle A7 centre (-31.1127, -31.1127) radius 2.5
  circle A8 centre (31.1127, -31.1127) radius 2.5
  dimension "d127" = 88
  dimension "d126" = 2.7
  dimension "d130" = 360
  dimension "d132" = 5
  dimension "d135" = 360
  constraints: 8 centre point, 2 coincident, 1 point on line, 21 other
  measures "d126" diameter of A0
  measures "d132" diameter of A5
extrude "押し出し24" cut sketch "スケッチ11" along normal blind 19.5 contours A0 | A2 | A3 | A4 | A5 | A6 | A7 | A8
extrude "押し出し25" cut sketch "スケッチ11" along normal through all contours A0 | A2 | A3 | A4
sketch "スケッチ12" plane through (0, 33.5, 0) normal (0, 1, 0) x (1, 0, 0)
  point P0 (0, 0)
sketch "スケッチ13" plane through (0, 0, 0) normal (0, 1, 0) x (-1, 0, 0)
  circle A0 centre (-31.1127, -31.1127) radius 1.35 projected
  circle A1 centre (-31.1127, 31.1127) radius 1.35 projected
  circle A2 centre (31.1127, -31.1127) radius 1.35 projected
  circle A3 centre (31.1127, 31.1127) radius 1.35 projected
  line L0 (11.3, -21.15) -> (11.3, -24.15) projected
  line L1 (11.3, -24.15) -> (8.95, -24.15) projected
  line L2 (8.95, -24.15) -> (8.95, -25) projected
  line L3 (8.95, -25) -> (14, -25) projected
  line L4 (14, -25) -> (14, -35.5) projected
  line L5 (14, -35.5) -> (-14, -35.5) projected
  line L6 (-14, -35.5) -> (-14, -25) projected
  line L7 (-14, -25) -> (-8.95, -25) projected
  line L8 (-8.95, -25) -> (-8.95, -24.15) projected
  line L9 (-8.95, -24.15) -> (-11.3, -24.15) projected
  line L10 (-11.3, -24.15) -> (-11.3, -21.15) projected
  line L11 (-11.3, -21.15) -> (-12.15, -21.15) projected
  line L12 (-12.15, -21.15) -> (-12.15, -14.85) projected
  line L13 (-12.15, -14.85) -> (-11.3, -14.85) projected
  line L14 (-11.3, -14.85) -> (-11.3, -12.85) projected
  line L15 (-11.3, -12.85) -> (-13.7, -12.85) projected
  line L16 (-13.7, -12.85) -> (-13.7, -20.15) projected
  line L17 (-13.7, -20.15) -> (-34, -20.15) projected
  line L18 (-34, -20.15) -> (-34, -13.1699) projected
  arc A4 (-35.3682, -12.85) -> (-34, -13.1699) centre (-34.02, -10.17) ccw projected
  line L19 (-35.3682, -12.85) -> (-36.7, -12.85) projected
  arc A5 (-36.7, 11.5182) -> (-36.7, 8.8218) centre (-34.02, 10.17) ccw projected
  line L20 (-36.7, 12.85) -> (-35.3682, 12.85) projected
  line L21 (-34, 13.1699) -> (-34, 20.15) projected
  line L22 (-34, 20.15) -> (-13.7, 20.15) projected
  line L23 (-13.7, 20.15) -> (-13.7, 12.85) projected
  line L24 (-13.7, 12.85) -> (-11.3, 12.85) projected
  line L25 (-11.3, 12.85) -> (-11.3, 14.85) projected
  line L26 (-11.3, 14.85) -> (-12.15, 14.85) projected
  line L27 (-12.15, 14.85) -> (-12.15, 21.15) projected
  line L28 (-12.15, 21.15) -> (-11.3, 21.15) projected
  line L29 (-11.3, 21.15) -> (-11.3, 24.15) projected
  line L30 (-11.3, 24.15) -> (-8.95, 24.15) projected
  line L31 (-8.95, 24.15) -> (-8.95, 25) projected
  line L32 (-8.95, 25) -> (-14, 25) projected
  line L33 (-14, 25) -> (-14, 35.5) projected
  line L34 (-14, 35.5) -> (14, 35.5) projected
  line L35 (14, 35.5) -> (14, 25) projected
  line L36 (14, 25) -> (8.95, 25) projected
  line L37 (8.95, 25) -> (8.95, 24.15) projected
  line L38 (8.95, 24.15) -> (11.3, 24.15) projected
  line L39 (11.3, 24.15) -> (11.3, 21.15) projected
  line L40 (11.3, 21.15) -> (12.15, 21.15) projected
  line L41 (12.15, 21.15) -> (12.15, 14.85) projected
  line L42 (12.15, 14.85) -> (11.3, 14.85) projected
  line L43 (11.3, 14.85) -> (11.3, 9.15) projected
  line L44 (11.3, 9.15) -> (12.15, 9.15) projected
  line L45 (12.15, 9.15) -> (12.15, 2.85) projected
  line L46 (12.15, 2.85) -> (11.3, 2.85) projected
  line L47 (11.3, 2.85) -> (11.3, -2.85) projected
  line L48 (11.3, -2.85) -> (12.15, -2.85) projected
  line L49 (12.15, -2.85) -> (12.15, -9.15) projected
  line L50 (12.15, -9.15) -> (11.3, -9.15) projected
  line L51 (11.3, -9.15) -> (11.3, -14.85) projected
  line L52 (11.3, -14.85) -> (12.15, -14.85) projected
  line L53 (12.15, -14.85) -> (12.15, -21.15) projected
  line L54 (12.15, -21.15) -> (11.3, -21.15) projected
  line L55 (14.85, -33.65) -> (14.85, 33.65) projected
  line L56 (14.85, 33.65) -> (29.15, 33.65) projected
  line L57 (29.15, 33.65) -> (29.15, 21.2895) projected
  line L58 (29.15, 21.2895) -> (37.55, 21.2895) projected
  line L59 (37.55, 21.2895) -> (37.55, 27.55) projected
  arc A6 (37.55, 27.55) -> (27.55, 37.55) centre (27.55, 27.55) ccw projected
  line L60 (27.55, 37.55) -> (-27.55, 37.55) projected
  arc A7 (-27.55, 37.55) -> (-37.55, 27.55) centre (-27.55, 27.55) ccw projected
  arc A8 (-37.55, -27.55) -> (-27.55, -37.55) centre (-27.55, -27.55) ccw projected
  line L61 (-27.55, -37.55) -> (27.55, -37.55) projected
  arc A9 (27.55, -37.55) -> (37.55, -27.55) centre (27.55, -27.55) ccw projected
  line L62 (37.55, -27.55) -> (37.55, -21.2895) projected
  line L63 (37.55, -21.2895) -> (29.15, -21.2895) projected
  line L64 (29.15, -21.2895) -> (29.15, -33.65) projected
  line L65 (29.15, -33.65) -> (27, -33.65) projected
  line L66 (27, -33.65) -> (27, -35) projected
  line L67 (27, -35) -> (17, -35) projected
  line L68 (17, -35) -> (17, -33.65) projected
  line L69 (17, -33.65) -> (14.85, -33.65) projected
  line L70 (-17.55, 24.15) -> (-17.55, 37.55)
  line L71 (-27.55, 37.55) -> (-27.55, 20.15)
  line L72 (-11.3, 24.15) -> (-17.55, 24.15)
  line L73 (-13.7, 12.85) -> (-13.7, -12.85)
  line L74 (-11.3, 12.85) -> (-11.3, 9.15)
  line L75 (-11.3, 9.15) -> (-12.15, 9.15)
  line L76 (-12.15, 9.15) -> (-12.15, -9.15)
  line L77 (-12.15, -9.15) -> (-11.3, -9.15)
  line L78 (-11.3, -9.15) -> (-11.3, -12.85)
  line L79 (-11.15, 0) -> (-11.15, 24) projected
  line L80 (-12, 3) -> (-12, 9) projected
  line L81 (-11.15, 3) -> (-12, 3) projected
  line L82 (-11.15, 0) -> (-11.15, -24) projected
  line L83 (-11.15, -3) -> (-12, -3) projected
  line L84 (-12, -3) -> (-12, -9) projected
  line L85 (-12, -9) -> (-11.15, -9) projected
  line L86 (-12.15, 2.85) -> (-11.3, 2.85)
  line L87 (-11.3, 2.85) -> (-11.3, -2.85)
  line L88 (-11.3, -2.85) -> (-12.15, -2.85)
  line L89 (-12, 9) -> (-11.15, 9) projected
  line L90 (55.4695, 0) -> (-55.4695, 0) construction
  line L91 (-17.55, -24.15) -> (-17.55, -37.55)
  line L92 (-27.55, -37.55) -> (-27.55, -20.15)
  line L93 (-11.3, -24.15) -> (-17.55, -24.15)
  line L94 (-22.55, 37.55) -> (-22.55, -37.55)
  line L95 (-17.55, 24.15) -> (-22.55, 24.15)
  line L96 (-17.55, -24.15) -> (-37.55, -24.15)
  line L97 (-22.55, 24.15) -> (-37.4, 24.15)
  line L98 (-34, -20.15) -> (-37.55, -20.15)
  line L99 (-34, 20.15) -> (-37.55, 20.15)
  line L100 (-27.55, 30.15) -> (-17.55, 30.15)
  line L101 (-27.55, 24.95) -> (-17.55, 24.95)
  line L102 (-27.55, 30.15) -> (-27.55, 24.95)
  line L103 (-17.55, 24.95) -> (-17.55, 30.15)
  line L104 (-17.55, 27.55) -> (-27.55, 27.55) construction
  line L105 (-27.55, -27.55) -> (-17.55, -27.55) construction
  line L106 (-27.55, -30.15) -> (-17.55, -30.15)
  line L107 (-27.55, -24.95) -> (-17.55, -24.95)
  line L108 (-37.55, 27.55) -> (-37.55, -27.55) projected
  line L109 (-36.7, -12.85) -> (-36.7, -11.5182) projected
  arc A10 (-36.7, -8.8218) -> (-36.7, -11.5182) centre (-34.02, -10.17) ccw projected
  line L110 (-36.7, -8.8218) -> (-36.7, 8.8218) projected
  line L111 (-36.7, 11.5182) -> (-36.7, 12.85) projected
  arc A11 (-34, 13.1699) -> (-35.3682, 12.85) centre (-34.02, 10.17) ccw projected
  point P0 (0, 0)
  point P1 (-27.55, 24.15)
  point P2 (-27.55, -24.15)
  point P3 (-22.55, 30.15)
  point P4 (-22.55, 24.95)
  point P5 (-22.55, -24.95)
  point P6 (-22.55, -30.15)
  point P7 (-37.55, -20.15)
  point P8 (-37.55, -24.15)
  point P9 (-11.3, 9.15)
  dimension "d142" = 10
  dimension "d143" = 0.15
  dimension "d144" = 0.15
  dimension "d145" = 0.15
  dimension "d146" = 0.15
  dimension "d147" = 0.15
  dimension "d148" = 0.15
  dimension "d150" = 5
  dimension "d153" = 5.2
  dimension "d155" = 5.2
  dimension "d162" = 10
  dimension "d163" = 10
  dimension "d164" = 2.6
  constraints: 58 end point, 21 point on line, 14 perpendicular, 6 horizontal, 4 vertical, 3 parallel, 3 symmetric about line, 2 midpoint, 1 collinear
  measures "d142" distance between parallel lines of L71 L70
  measures "d143" distance between parallel lines of L76 L80
  measures "d144" distance between parallel lines of L87 L79
  measures "d145" distance between parallel lines of L86 L81
  measures "d146" distance between parallel lines of L83 L88
  measures "d147" distance between parallel lines of L75 L89
  measures "d148" distance between parallel lines of L77 L85
  measures "d150" distance between parallel lines of L94 L91
  measures "d153" distance between parallel lines of L100 L101
  measures "d155" distance between parallel lines of L106 L107
  measures "d162" distance between parallel lines of L60 L104
  measures "d163" distance between parallel lines of L61 L105
  measures "d164" distance between parallel lines of L106 L105
extrude "押し出し26" cut sketch "スケッチ13" against normal blind 10 from surface at 33.5 contours L93 L96 L94 L17 L16 L15 L14 L13 L12 L11 L10 | L96 L92 L17 L94 | L96 L108 L98 L17 L92 | L92 A8 L108 L96 | L94 L95 L72 L29 L28 L27 L26 L25 L24 L23 L22 | L22 L71 L97 L94 | L15 L73 L24 L74 L75 L76 L77 L78 | L22 L99 L108 A7 L71 | L76 L86 L87 L88
extrude "押し出し27" cut sketch "スケッチ13" against normal blind 7.8 from surface at 33.5 contours L91 L106 L94 L107 | L94 L100 L70 L101
sketch "スケッチ14" plane through (27.55, 33.5, 37.55) normal (1, 0, 0) x (0, 0, -1)
  line L0 (0, 0) -> (0, -10) projected
  line L1 (0, 0) -> (13.4, 0) projected
  line L2 (0, -10) -> (13.4, -10) projected
  line L3 (13.4, -10) -> (13.4, 0) projected
  line L4 (0, 0) -> (13.4, -10) construction
  line L5 (0, -10) -> (13.4, 0) construction
  line L6 (37.55, -40.2) -> (37.55, 6.7) construction
  line L7 (0, -5) -> (13.4, -5) construction
  circle A0 centre (10, -5) radius 1.35
  circle A1 centre (65.1, -5) radius 1.35
  point P0 (37.55, -33.5)
  dimension "d165" = 2.7
  dimension "d166" = 10
  constraints: 6 end point, 2 centre point, 2 midpoint, 1 point on line, 1 symmetric about line, 1 other
  measures "d165" diameter of A0
  measures "d166" distance from line of L0 A0.centre
extrude "押し出し29" cut sketch "スケッチ14" against normal up to surface (5 mm away) contours A0 | A1
extrude "押し出し30" cut sketch "スケッチ1" along normal up to surface (33.5 mm away) contours L106 L56 L64 L62 | L35 L37 L12 L109 | L64 L56 L66 L62 | L35 L39 L12 L37 | L66 L56 L107 L62 | L35 L108 L12 L39
extrude "押し出し31" cut sketch "スケッチ1" along normal up to surface (33.5 mm away) contours L112 L113 L56 L106 | L109 L12 L117 L116 | L107 L56 L110 L111 | L115 L114 L12 L108
extrude "押し出し33" cut sketch "スケッチ1" against normal blind 2 from surface at 14 contours L120 L126 L22 L123 | L123 L24 L127 L121 | L22 L126 L118 L123 | L120 L122 L22 L126 | L123 L119 L127 L24 | L127 L24 L122 L121 | L118 L126 L96 L127 L119 L123 A15 | L22 L122 L118 L126 | L127 L119 L122 L24 | A15 L123 | L118 L122 L119 L127 L95 L94 L93 L126 | L93 L94 L95 L96
extrude "押し出し34" cut sketch "スケッチ1" against normal blind 4 from surface at 14 contours L118 L88 A15 L119 L7 | L118 L123 A15 L88 | L88 A15 L123 L119 | A15 L123 L88 A14 | L88 A14 A15 | A14 L88 | L88 A14
extrude "押し出し35" cut sketch "スケッチ6" against normal blind 4 from surface at 14 contours L4 L21 L6 L20
extrude "押し出し36" cut sketch "スケッチ1" along normal blind 14 contours L118 L123 A15 L88 | L22 L126 L118 L123 | L88 A15 L123 L119 | L123 L119 L127 L24 | A15 L123 L88 A14 | L118 L126 L96 L127 L119 L123 A15 | L22 L122 L118 L126 | L127 L119 L122 L24 | A14 L88 | A15 L123 | L118 L122 L119 L127 L95 L94 L93 L126 | L118 L86 L119 L122 picked at (-32.5953, 0.4408)
fillet "フィレット2" radius 2.3 4 edges at (33.85, 7, 8.17) (13.85, 7, 8.17) (13.85, 7, -8.17) (33.85, 7, -8.17)
extrude "押し出し37" add sketch "スケッチ1" along normal up to surface (2 mm away) from surface at 12 contours L120 L126 L22 L123 | L123 L24 L127 L121 | L120 L122 L22 L126 | L127 L24 L122 L121
ref_plane "作業平面3" through (23.85, 0, -2.4571) normal (-1, 0, 0) x (0, 0, 1)
sketch "スケッチ17" plane through (23.85, 0, -2.4571) normal (-1, 0, 0) x (0, 0, 1)
  line L0 (-3.4129, 10) -> (8.3271, 10) projected
  line L1 (10.6271, 10) -> (8.3271, 10) projected
  line L2 (-5.7129, 10) -> (10.6271, 10) projected
  line L3 (-3.4129, 10) -> (-5.7129, 10) projected
  line L4 (2.4571, 10) -> (2.4571, -12.9308)
  line L5 (8.3271, 14) -> (-3.4129, 14) projected
  line L6 (2.4571, 10) -> (2.4571, 14)
  line L7 (10.6271, 0) -> (15.1571, 0) projected
  line L8 (8.3271, 0) -> (10.6271, 0) projected
  line L9 (-3.4129, 0) -> (8.3271, 0) projected
  line L10 (-1.5429, 0) -> (6.4571, 0) projected
  line L11 (6.4571, 0) -> (6.4571, 14)
  line L12 (-1.5429, 0) -> (-1.5429, 14)
  line L13 (6.4571, 14) -> (11.9525, -6.5089)
  line L14 (-1.5429, 14) -> (-7.0835, -6.6778)
  line L15 (6.4571, 10) -> (10.9698, -6.8416)
  line L16 (-1.5429, 10) -> (-6.0448, -6.8015)
  line L17 (-5.7129, 0) -> (-3.4129, 0) projected
  line L18 (-10.2429, 0) -> (-5.7129, 0) projected
  point P0 (2.4571, 0)
  dimension "d197" = 15
  dimension "d198" = 15
  constraints: 16 end point, 6 point on line, 2 midpoint, 2 parallel, 2 perpendicular, 1 vertical
  measures "d197" angle of L4 L13
  measures "d198" angle of L4 L14
